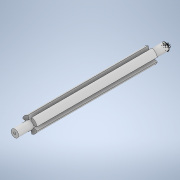
# Autodesk Inventor part: Nicoles_Roomba_Blade_Axle
Saved by Autodesk Inventor 2021 (Build 250183000, 183)
## iProperties
Created: 2021-03-31
Part Number: Nicoles_Roomba_Blade_Axle
Material: Generic
Document SubType Name: Modeling
Designer: saipr
Density: 1 g/cm^3
Appearance: Default
Author: saipr
Autodesk Inventor part; units mm, degrees
ref_plane "YZ Plane" through (0, 0, 0) normal (1, 0, 0) x (0, 1, 0)
ref_plane "XZ Plane" through (0, 0, 0) normal (0, 1, 0) x (-1, 0, 0)
ref_plane "XY Plane" through (0, 0, 0) normal (0, 0, 1) x (1, 0, 0)
sketch "Sketch1" plane through (0, 0, 0) normal (0, 0, 1) x (1, 0, 0)
  circle A0 centre (0, 0) radius 6.35
  line L0 (-1.5875, -1.5875) -> (1.5875, -1.5875)
  line L1 (1.5875, -1.5875) -> (1.5875, 1.5875)
  line L2 (1.5875, 1.5875) -> (-1.5875, 1.5875)
  line L3 (-1.5875, 1.5875) -> (-1.5875, -1.5875)
  line L4 (-1.5875, -1.5875) -> (1.5875, 1.5875) construction
  line L5 (1.5875, -1.5875) -> (-1.5875, 1.5875) construction
  dimension "d0" = 12.7
  dimension "d3" = 3.175
  dimension "d4" = 3.175
  constraints: 12 end point, 2 midpoint, 2 parallel, 1 centre point, 1 coincident, 1 horizontal, 1 perpendicular
  measures "d0" diameter of A0
  measures "d3" distance of L2.end L1.end
  measures "d4" distance of L1.end L0.end
extrude "Extrusion1" add sketch "Sketch1" along normal blind 254 contours A0 | L3 L2 L1 L0
extrude "Extrusion2" cut sketch "Sketch1" along normal blind 254 contours L3 L2 L1 L0
ref_plane "Work Plane1" through (0, 0, 25.4) normal (0, 0, -1) x (-1, 0, 0)
sketch "Sketch2" plane through (0, 0, 25.4) normal (0, 0, -1) x (-1, 0, 0)
  circle A0 centre (0, 0) radius 10.16
  line L0 (0, 0) -> (-12.2827, 3.2288)
  circle A1 centre (0, 0) radius 6.35 projected
  line L1 (-12.2827, -3.2288) -> (0, 0)
  arc A2 (-3.2288, 12.2827) -> (-12.2827, 3.2288) centre (0, 0) ccw
  arc A3 (12.2827, 3.2288) -> (3.2288, 12.2827) centre (0, 0) ccw
  arc A4 (-12.2827, -3.2288) -> (-3.2288, -12.2827) centre (0, 0) ccw
  arc A5 (3.2288, -12.2827) -> (12.2827, -3.2288) centre (0, 0) ccw
  line L2 (0, 0) -> (-3.2288, -12.2827)
  line L3 (3.2288, -12.2827) -> (0, 0)
  line L4 (0, 0) -> (12.2827, -3.2288)
  line L5 (12.2827, 3.2288) -> (0, 0)
  line L6 (0, 0) -> (3.2288, 12.2827)
  line L7 (-3.2288, 12.2827) -> (0, 0)
  point P0 (-1.6144, -6.1414)
  point P1 (-6.1414, -1.6144)
  point P2 (6.1414, -1.6144)
  point P3 (1.6144, -6.1414)
  point P4 (1.6144, 6.1414)
  point P5 (6.1414, 1.6144)
  point P6 (-6.1414, 1.6144)
  point P7 (-1.6144, 6.1414)
  dimension "d11" = 20.32
  dimension "d20" = 360
  constraints: 16 end point, 8 point on circle, 5 centre point, 2 coincident, 25 other
  measures "d11" diameter of A0
extrude "Extrusion4" add sketch "Sketch2" against normal blind 203.2 contours L5 A1 L6 A0 | A0 L6 A3 L5 | L4 A5 L3 A0 | A0 L3 A1 L4 | L7 A1 L0 A0 | A0 L0 A2 L7 | L2 A4 L1 A0 | A0 L1 A1 L2
body "Solid1"
